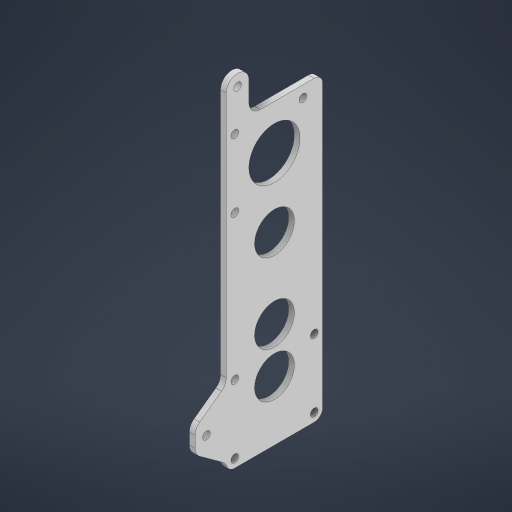
# Autodesk Inventor part: winch plate
Saved by Autodesk Inventor 2024 (Build 280153000, 153)
## iProperties
Created: 2024-03-28
Part Number: winch plate
Material: Generic
Document SubType Name: Modeling
Designer: Andrew
Density: 1 g/cm^3
Appearance: Default
Author: Andrew
Autodesk Inventor part; units mm, degrees
ref_plane "YZ Plane" through (0, 0, 0) normal (1, 0, 0) x (0, 1, 0)
ref_plane "XZ Plane" through (0, 0, 0) normal (0, 1, 0) x (-1, 0, 0)
ref_plane "XY Plane" through (0, 0, 0) normal (0, 0, 1) x (1, 0, 0)
sketch "Sketch1" plane through (0, 0, 0) normal (1, 0, 0) x (0, 1, 0)
  circle A0 centre (-31.75, 44.45) radius 11.1125
  circle A1 centre (-76.2, 44.45) radius 11.1125
  circle A2 centre (-101.6, 44.45) radius 11.1125
  line L0 (-130.175, 71.4375) -> (-92.075, 71.4375)
  arc A3 (-130.175, 71.4375) -> (-134.9375, 66.675) centre (-130.175, 66.675) ccw
  arc A4 (26.9875, 17.4625) -> (31.75, 22.225) centre (26.9875, 22.225) ccw
  line L1 (-130.175, 17.4625) -> (-92.075, 17.4625)
  circle A5 centre (25.4, 28.575) radius 2.1082
  circle A6 centre (-92.075, 66.675) radius 2.1082
  line L2 (31.75, 66.675) -> (31.75, 22.225)
  circle A7 centre (-92.075, 22.225) radius 2.1082
  arc A8 (-134.9375, 22.225) -> (-130.175, 17.4625) centre (-130.175, 22.225) ccw
  circle A9 centre (-130.175, 66.675) radius 2.1082
  line L3 (-134.9375, 66.675) -> (-134.9375, 22.225)
  circle A10 centre (-130.175, 22.225) radius 2.1082
  line L4 (-92.075, 71.4375) -> (26.9875, 71.4375)
  arc A11 (31.75, 66.675) -> (26.9875, 71.4375) centre (26.9875, 66.675) ccw
  circle A12 centre (26.9875, 66.675) radius 2.1345
  line L5 (-92.075, 17.4625) -> (26.9875, 17.4625)
  line L6 (26.9875, 66.675) -> (-17.4625, 66.675)
  line L7 (-17.4625, 66.675) -> (-11.1125, 66.675)
  line L8 (-17.4625, 66.675) -> (-23.8125, 66.675)
  circle A13 centre (-11.1125, 66.675) radius 2.1345
  line L9 (26.9875, 44.45) -> (6.6675, 44.45)
  circle A14 centre (6.6675, 44.45) radius 14.2875
  line L10 (-130.175, 22.225) -> (-92.075, 22.225)
  line L11 (-111.125, 22.225) -> (-111.125, 6.35)
  circle A15 centre (-111.125, 6.35) radius 2.1336
  line L12 (-111.125, 6.35) -> (-111.125, 0)
  line L13 (-111.125, 0) -> (-117.475, 0)
  line L14 (-111.125, 0) -> (-104.775, 0)
  line L15 (-117.475, 0) -> (-130.175, 17.4625)
  line L16 (-104.775, 0) -> (-92.075, 17.4625)
  line L17 (-130.175, 66.675) -> (-92.075, 66.675)
  line L18 (-111.125, 66.675) -> (-111.125, 82.55)
  circle A16 centre (-111.125, 82.55) radius 2.1336
  line L19 (-111.125, 82.55) -> (-111.125, 88.9)
  line L20 (-111.125, 88.9) -> (-117.475, 88.9)
  line L21 (-117.475, 88.9) -> (-104.775, 88.9)
  line L22 (-104.775, 88.9) -> (-92.075, 71.4375)
  line L23 (-117.475, 88.9) -> (-130.175, 71.4375)
  line L24 (26.9875, 71.4375) -> (55.5625, 71.4375)
  line L25 (55.5625, 71.4375) -> (55.5625, 58.7375)
  line L26 (55.5625, 58.7375) -> (31.75, 58.7375)
  line L27 (55.5625, 65.0875) -> (49.2125, 65.0875)
  circle A17 centre (49.2125, 65.0875) radius 2.1336
  point P0 (0, 0)
  point P1 (26.9875, 71.4375)
  dimension "d2" = 6.35
  dimension "d3" = 6.35
  dimension "d4" = 44.45
  dimension "d5" = 20.32
  dimension "d6" = 28.575
  dimension "d7" = 4.2672
  dimension "d8" = 6.35
  dimension "d9" = 6.35
  dimension "d10" = 6.35
  dimension "d11" = 15.875
  dimension "d12" = 4.2672
  dimension "d13" = 6.35
  dimension "d14" = 6.35
  dimension "d15" = 12.7
  dimension "d21" = 28.575
  dimension "d22" = 6.35
  dimension "d23" = 4.2672
  constraints: 56 end point, 18 centre point, 9 horizontal, 8 point on circle, 5 coincident, 5 point on line, 3 midpoint, 3 vertical, 2 perpendicular, 1 tangent, 3 other
  measures "d2" distance of L6.end L7.end
  measures "d3" distance of L6.end L8.end
  measures "d4" distance of L6.start L6.end
  measures "d5" distance of L9.start L9.end
  measures "d6" diameter of A14
  measures "d7" diameter of A15
  measures "d8" distance of L12.start L12.end
  measures "d9" distance of L12.end L13.end
  measures "d10" distance of L12.end L14.end
  measures "d11" distance of L18.start L18.end
  measures "d12" diameter of A16
  measures "d13" distance of L19.start L19.end
  measures "d14" distance of L19.end L20.end
  measures "d15" distance of L20.end L21.end
  measures "d21" distance of L24.start L24.end
  measures "d22" distance of L27.start L27.end
  measures "d23" diameter of A17
extrude "Extrusion1" add sketch "Sketch1" along normal blind 3.175 contours L23 L20 L19 A16 L18 L0 | L0 L4 A11 L2 A4 L5 L1 A8 L3 A3 | L18 A16 L19 L21 L22 L0 | L24 L25 L26 L2 A11
fillet "Fillet1" radius 6.35 4 edges at (1.5875, -130.175, 71.4375) (1.5875, -117.475, 88.9) (1.5875, -104.775, 88.9) (1.5875, -92.075, 71.4375)
fillet "Fillet3" radius 6.35 3 edges at (1.5875, 31.75, 58.7375) (1.5875, 55.5625, 58.7375) (1.5875, 55.5625, 71.4375)
body "Solid1"
